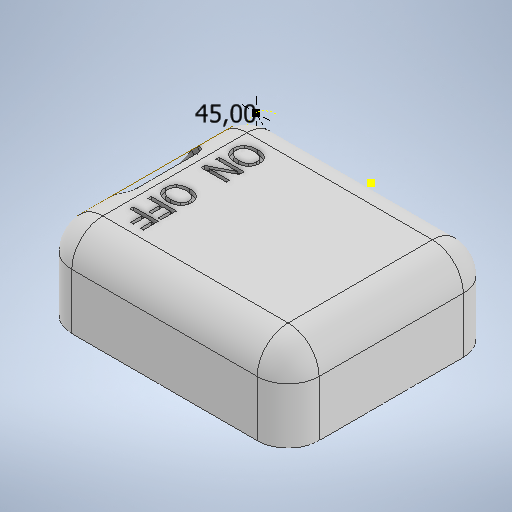
# Autodesk Inventor part: PCB_Deckel
Saved by Autodesk Inventor 2025.2 (Build 292293000, 293)
## iProperties
Created: 2024-11-12
Part Number: PCB_Deckel
Material: Generic
Document SubType Name: Modeling
Designer: matss
Density: 1 g/cm^3
Appearance: Default
Author: matss
Autodesk Inventor part; units mm, degrees
ref_plane "YZ Plane" through (0, 0, 0) normal (1, 0, 0) x (0, 1, 0)
ref_plane "XZ Plane" through (0, 0, 0) normal (0, 1, 0) x (-1, 0, 0)
ref_plane "XY Plane" through (0, 0, 0) normal (0, 0, 1) x (1, 0, 0)
sketch "Sketch1" plane through (0, 0, 0) normal (0, 1, 0) x (-1, 0, 0)
  line L0 (22.5, 22.5) -> (-22.5, 22.5)
  line L1 (-27.5, 17.5) -> (-27.5, -17.5)
  line L2 (-22.5, -22.5) -> (22.5, -22.5)
  line L3 (27.5, -17.5) -> (27.5, 17.5)
  arc A0 (27.5, 17.5) -> (22.5, 22.5) centre (22.5, 17.5) ccw
  arc A1 (22.5, -22.5) -> (27.5, -17.5) centre (22.5, -17.5) ccw
  arc A2 (-27.5, -17.5) -> (-22.5, -22.5) centre (-22.5, -17.5) ccw
  arc A3 (-22.5, 22.5) -> (-27.5, 17.5) centre (-22.5, 17.5) ccw
  line L4 (30, 17.5) -> (30, -17.5)
  arc A4 (22.5, -25) -> (30, -17.5) centre (22.5, -17.5) ccw
  line L5 (22.5, -25) -> (-22.5, -25)
  arc A5 (-30, -17.5) -> (-22.5, -25) centre (-22.5, -17.5) ccw
  line L6 (-30, -17.5) -> (-30, 17.5)
  arc A6 (-22.5, 25) -> (-30, 17.5) centre (-22.5, 17.5) ccw
  line L7 (-22.5, 25) -> (22.5, 25)
  arc A7 (30, 17.5) -> (22.5, 25) centre (22.5, 17.5) ccw
  point P0 (0, 0)
  point P1 (27.5, 22.5)
  point P2 (27.5, -22.5)
  point P3 (0, 22.5)
  point P4 (27.5, 0)
  dimension "d0" = 45
  dimension "d1" = 55
  dimension "d2" = 5
  dimension "d3" = 2.5
  constraints: 16 end point, 16 point on circle, 8 centre point, 8 tangent, 4 parallel, 4 point on line, 3 equal radius, 2 midpoint, 2 perpendicular, 1 horizontal, 1 horizontal alignment, 1 vertical alignment, 7 other
  measures "d0" distance of point (27.5, -22.5) point (27.5, 22.5)
  measures "d1" distance between parallel lines of L1 L3
  measures "d2" radius of A0
  measures "d3" distance between parallel lines of L3 L4
extrude "Extrusion1" add sketch "Sketch1" along normal blind 3 contours A0 L3 A1 L2 A2 L1 A3 L0 | L4 A4 L5 A5 L6 A6 L7 A7
extrude "Extrusion2" add sketch "Sketch1" against normal blind 18
fillet "Fillet1" radius 5 8 edges at (26.0355, 0, 21.0355) (0, 0, 22.5) (-26.0355, 0, 21.0355) (-27.5, 0, 0) (-26.0355, 0, -21.0355) (0, 0, -22.5) (26.0355, 0, -21.0355) (27.5, 0, 0)
fillet "Fillet2" radius 7.5 8 edges at (-27.8033, 3, -22.8033) (-30, 3, 0) (-27.8033, 3, 22.8033) (0, 3, 25) (27.8033, 3, 22.8033) (30, 3, 0) (27.8033, 3, -22.8033) (0, 3, -25)
sketch "Sketch2" plane through (22.5, -18, -25) normal (0, 0, -1) x (-1, 0, 0)
  arc A0 (52.5, 13.5) -> (45, 21) centre (45, 13.5) ccw construction
  line L0 (45, 13.5) -> (50.3033, 18.8033) construction
  line L1 (45, 13.5) -> (52.5, 13.5) construction
  point P0 (22.5, 18)
  point P1 (50.3033, 18.8033)
  point P2 (50.3033, 18.8033)
  dimension "d10" = 45
  constraints: 4 end point, 2 point on circle, 1 coincident
  measures "d10" angle of L1 L0
ref_plane "Work Plane1" through (-27.8033, 0.8033, -25) normal (-0.7071068, 0.7071068, 0) x (-0.7071068, -0.7071068, 0)
sketch "Sketch3" plane through (-27.8033, 0.8033, -25) normal (-0.7071068, 0.7071068, 0) x (-0.7071068, -0.7071068, 0)
  line L0 (-5.3033, 42.5) -> (-5.3033, 7.5) construction
  line L1 (5.3033, 7.5) -> (5.3033, 42.5) construction
  line L2 (-3.75, 15) -> (3.75, 15)
  line L3 (3.75, 15) -> (3.75, 35)
  line L4 (3.75, 35) -> (-3.75, 35)
  line L5 (-3.75, 35) -> (-3.75, 15)
  line L6 (-5.3033, 25) -> (5.3033, 25) construction
  point P0 (-19.0919, 25)
  point P1 (-3.75, 25)
  point P2 (0, 15)
  point P3 (0, 25)
  dimension "d11" = 7.5
  dimension "d12" = 20
  constraints: 10 end point, 5 midpoint, 2 parallel, 1 horizontal, 1 perpendicular, 1 point on line, 1 vertical alignment
  measures "d11" distance between parallel lines of L3 L5
  measures "d12" distance of L4.end L2.start
extrude "Extrusion3" cut sketch "Sketch3" against normal blind 10
fillet "Fillet3" radius 2.75 4 edges at (-23.0689, 1.3722, -10) (-23.0689, 1.3722, 10) (-28.6204, -3.6829, 10) (-28.6204, -3.6829, -10)
sketch "Sketch4" plane through (0, 3, 0) normal (0, 1, 0) x (1, 0, 0)
  line L0 (-22.5, -17.5) -> (-22.5, 17.5) projected
  line L1 (-14.5, 15.5) -> (-14.5, 4.589) construction
  line L2 (-14.5, 4.589) -> (-24.5824, 4.589) construction
  line L3 (-24.5824, 4.589) -> (-24.5824, 15.5) construction
  line L4 (-24.5824, 15.5) -> (-14.5, 15.5) construction
  line L5 (-14.5, -0.9745) -> (-14.5, -15.5) construction
  line L6 (-14.5, -15.5) -> (-17.6148, -15.5) construction
  line L7 (-17.6148, -15.5) -> (-17.6148, -0.9745) construction
  line L8 (-17.6148, -0.9745) -> (-14.5, -0.9745) construction
  line L9 (-22.5, 17.5) -> (22.5, 17.5) projected
  line L10 (22.5, -17.5) -> (-22.5, -17.5) projected
  spline S0 degree 2 poles (-15.325, 10.5698) (-15.7301, 10.224) (-16.9157, 9.8387) (-17.6764, 9.8387) knots 0 0 0 1 2 2 2
  spline S1 degree 2 poles (-17.6764, 9.8387) (-18.4174, 9.8387) (-19.6179, 10.2142) (-20.023, 10.5698) knots 0 0 0 1 2 2 2
  spline S2 degree 2 poles (-20.023, 10.5698) (-20.4478, 10.9453) (-20.8529, 11.9382) (-20.8529, 12.536) knots 0 0 0 1 2 2 2
  spline S3 degree 2 poles (-20.8529, 12.536) (-20.8529, 13.1535) (-20.433, 14.1415) (-20.023, 14.5021) knots 0 0 0 1 2 2 2
  spline S4 degree 2 poles (-20.023, 14.5021) (-19.6179, 14.8529) (-18.4273, 15.2283) (-17.6764, 15.2283) knots 0 0 0 1 2 2 2
  spline S5 degree 2 poles (-17.6764, 15.2283) (-16.9107, 15.2283) (-15.7449, 14.8479) (-15.325, 14.4972) knots 0 0 0 1 2 2 2
  spline S6 degree 2 poles (-15.325, 14.4972) (-14.9199, 14.1415) (-14.5, 13.1485) (-14.5, 12.536) knots 0 0 0 1 2 2 2
  spline S7 degree 2 poles (-14.5, 12.536) (-14.5, 11.9135) (-14.9347, 10.9156) (-15.325, 10.5698) knots 0 0 0 1 2 2 2
  spline S8 degree 2 poles (-17.6764, 10.6835) (-17.0738, 10.6835) (-16.1401, 10.9453) (-15.8338, 11.1824) knots 0 0 0 1 2 2 2
  spline S9 degree 2 poles (-15.8338, 11.1824) (-15.5176, 11.4245) (-15.2015, 12.1062) (-15.2015, 12.531) knots 0 0 0 1 2 2 2
  spline S10 degree 2 poles (-15.2015, 12.531) (-15.2015, 12.9707) (-15.5078, 13.6327) (-15.8338, 13.8846) knots 0 0 0 1 2 2 2
  spline S11 degree 2 poles (-15.8338, 13.8846) (-16.145, 14.1267) (-17.0836, 14.3836) (-17.6764, 14.3836) knots 0 0 0 1 2 2 2
  spline S12 degree 2 poles (-17.6764, 14.3836) (-18.8769, 14.3836) (-20.1514, 13.3758) (-20.1514, 12.531) knots 0 0 0 1 2 2 2
  spline S13 degree 2 poles (-20.1514, 12.531) (-20.1514, 11.6863) (-18.8769, 10.6835) (-17.6764, 10.6835) knots 0 0 0 1 2 2 2
  line L11 (-20.7244, 4.5875) -> (-20.7244, 5.4964)
  line L12 (-20.7244, 5.4964) -> (-15.4682, 8.1937)
  line L13 (-15.4682, 8.1937) -> (-20.7244, 8.1937)
  line L14 (-20.7244, 8.1937) -> (-20.7244, 8.9495)
  line L15 (-20.7244, 8.9495) -> (-14.6284, 8.9495)
  line L16 (-14.6284, 8.9495) -> (-14.6284, 7.7985)
  line L17 (-14.6284, 7.7985) -> (-19.4549, 5.3433)
  line L18 (-19.4549, 5.3433) -> (-14.6284, 5.3433)
  line L19 (-14.6284, 5.3433) -> (-14.6284, 4.5875)
  line L20 (-14.6284, 4.5875) -> (-20.7244, 4.5875)
  spline S14 degree 2 poles (-15.325, -5.9046) (-15.7301, -6.2504) (-16.9157, -6.6357) (-17.6764, -6.6357) knots 0 0 0 1 2 2 2
  spline S15 degree 2 poles (-17.6764, -6.6357) (-18.4174, -6.6357) (-19.6179, -6.2603) (-20.023, -5.9046) knots 0 0 0 1 2 2 2
  spline S16 degree 2 poles (-20.023, -5.9046) (-20.4478, -5.5292) (-20.8529, -4.5362) (-20.8529, -3.9385) knots 0 0 0 1 2 2 2
  spline S17 degree 2 poles (-20.8529, -3.9385) (-20.8529, -3.321) (-20.433, -2.333) (-20.023, -1.9724) knots 0 0 0 1 2 2 2
  spline S18 degree 2 poles (-20.023, -1.9724) (-19.6179, -1.6216) (-18.4273, -1.2462) (-17.6764, -1.2462) knots 0 0 0 1 2 2 2
  spline S19 degree 2 poles (-17.6764, -1.2462) (-16.9107, -1.2462) (-15.7449, -1.6266) (-15.325, -1.9773) knots 0 0 0 1 2 2 2
  spline S20 degree 2 poles (-15.325, -1.9773) (-14.9199, -2.333) (-14.5, -3.3259) (-14.5, -3.9385) knots 0 0 0 1 2 2 2
  spline S21 degree 2 poles (-14.5, -3.9385) (-14.5, -4.5609) (-14.9347, -5.5588) (-15.325, -5.9046) knots 0 0 0 1 2 2 2
  spline S22 degree 2 poles (-17.6764, -5.791) (-17.0738, -5.791) (-16.1401, -5.5292) (-15.8338, -5.2921) knots 0 0 0 1 2 2 2
  spline S23 degree 2 poles (-15.8338, -5.2921) (-15.5176, -5.05) (-15.2015, -4.3683) (-15.2015, -3.9434) knots 0 0 0 1 2 2 2
  spline S24 degree 2 poles (-15.2015, -3.9434) (-15.2015, -3.5038) (-15.5078, -2.8418) (-15.8338, -2.5899) knots 0 0 0 1 2 2 2
  spline S25 degree 2 poles (-15.8338, -2.5899) (-16.145, -2.3478) (-17.0836, -2.0909) (-17.6764, -2.0909) knots 0 0 0 1 2 2 2
  spline S26 degree 2 poles (-17.6764, -2.0909) (-18.8769, -2.0909) (-20.1514, -3.0987) (-20.1514, -3.9434) knots 0 0 0 1 2 2 2
  spline S27 degree 2 poles (-20.1514, -3.9434) (-20.1514, -4.7882) (-18.8769, -5.791) (-17.6764, -5.791) knots 0 0 0 1 2 2 2
  line L21 (-15.3497, -11.1707) -> (-15.3497, -8.3351)
  line L22 (-15.3497, -8.3351) -> (-17.0688, -8.3351)
  line L23 (-17.0688, -8.3351) -> (-17.0688, -11.0521)
  line L24 (-17.0688, -11.0521) -> (-17.7901, -11.0521)
  line L25 (-17.7901, -11.0521) -> (-17.7901, -8.3351)
  line L26 (-17.7901, -8.3351) -> (-20.7244, -8.3351)
  line L27 (-20.7244, -8.3351) -> (-20.7244, -7.525)
  line L28 (-20.7244, -7.525) -> (-14.6284, -7.525)
  line L29 (-14.6284, -7.525) -> (-14.6284, -11.1707)
  line L30 (-14.6284, -11.1707) -> (-15.3497, -11.1707)
  line L31 (-15.3497, -15.5426) -> (-15.3497, -12.707)
  line L32 (-15.3497, -12.707) -> (-17.0688, -12.707)
  line L33 (-17.0688, -12.707) -> (-17.0688, -15.4241)
  line L34 (-17.0688, -15.4241) -> (-17.7901, -15.4241)
  line L35 (-17.7901, -15.4241) -> (-17.7901, -12.707)
  line L36 (-17.7901, -12.707) -> (-20.7244, -12.707)
  line L37 (-20.7244, -12.707) -> (-20.7244, -11.8969)
  line L38 (-20.7244, -11.8969) -> (-14.6284, -11.8969)
  line L39 (-14.6284, -11.8969) -> (-14.6284, -15.5426)
  line L40 (-14.6284, -15.5426) -> (-15.3497, -15.5426)
  point P0 (0, 0)
  point P1 (-24.4411, 7.25)
  point P2 (-27.0488, 10)
  point P3 (-27.0488, -10)
  dimension "d16" = 2
  dimension "d17" = 2
  dimension "d18" = 8
  constraints: 1 vertical alignment, 4 other
  measures "d16" distance from line of L9 L1.start
  measures "d17" distance from line of L10 L5.end
  measures "d18" distance from line of L0 L1.start
emboss "Emboss1" sketch "Sketch4" operation cut depth 1 direction (0, -1, 0)
body "Solid1"
